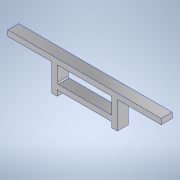
# Autodesk Inventor part: waist1.
Saved by Autodesk Inventor 2022 (Build 260153000, 153)
## iProperties
Created: 2022-10-16
Part Number: waist1.
Material: アルミニウム 6061
Document SubType Name: Modeling
Designer: haya
Density: 2.7 g/cm^3
Appearance: アルミニウム - フラット
Mass: 29.7232 g
Surface Area: 65.8455 cm^2
Volume: 11.0086 cm^3
Author: haya
Autodesk Inventor part; units mm, degrees
ref_plane "YZ Plane" through (0, 0, 0) normal (1, 0, 0) x (0, 1, 0)
ref_plane "XZ Plane" through (0, 0, 0) normal (0, 1, 0) x (-1, 0, 0)
ref_plane "XY Plane" through (0, 0, 0) normal (0, 0, 1) x (1, 0, 0)
sketch "スケッチ1" plane through (0, 0, 0) normal (0, 0, 1) x (1, 0, 0)
  line L0 (130, 25) -> (130, 30)
  line L1 (130, 30) -> (-10, 30)
  line L2 (-10, 30) -> (-10, 25)
  line L3 (60, 30) -> (60, 0) construction
  line L4 (85, 0) -> (85, 5)
  line L5 (85, 5) -> (35, 5)
  line L6 (35, 5) -> (35, 0)
  line L7 (30, 0) -> (35, 0)
  line L8 (85, 0) -> (90, 0)
  line L9 (30, 0) -> (30, 25)
  line L10 (30, 25) -> (-10, 25)
  line L11 (90, 0) -> (90, 25)
  line L12 (90, 25) -> (130, 25)
  dimension "d2" = 50
  dimension "d4" = 5
  dimension "d5" = 5
  dimension "d6" = 5
  dimension "d7" = 140
  dimension "d8" = 30
  constraints: 26 end point, 5 parallel, 2 horizontal, 2 perpendicular, 1 collinear, 1 midpoint, 2 other
  measures "d2" distance of L4.end L5.end
  measures "d4" distance between parallel lines of L8 L5
  measures "d5" distance between parallel lines of L10 L1
  measures "d6" distance between parallel lines of L9 L6
  measures "d7" distance of L0.end L1.end
  measures "d8" distance between parallel lines of L1 L7
extrude "押し出し1" add sketch "スケッチ1" along normal blind 10
sketch "スケッチ2" plane through (0, 0, 0) normal (0, 0, -1) x (-1, 0, 0)
  line L0 (-85, 10) -> (-35, 10)
  line L1 (-35, 10) -> (-35, 25)
  line L2 (-35, 25) -> (-85, 25)
  line L3 (-85, 25) -> (-85, 10)
  line L4 (-90, 0) -> (-90, 25) projected
  line L5 (-85, 0) -> (-90, 0) projected
  line L6 (-85, 5) -> (-85, 0) projected
  line L7 (-35, 5) -> (-85, 5) projected
  line L8 (-35, 0) -> (-35, 5) projected
  line L9 (-30, 0) -> (-35, 0) projected
  line L10 (-30, 25) -> (-30, 0) projected
  line L11 (10, 25) -> (-30, 25) projected
  line L12 (10, 30) -> (10, 25) projected
  line L13 (-130, 30) -> (10, 30) projected
  line L14 (-130, 25) -> (-130, 30) projected
  line L15 (-90, 25) -> (-130, 25) projected
  line L16 (-130, 30) -> (10, 30) projected
  line L17 (-60, 30) -> (-60, 5) construction
  line L18 (-35, 5) -> (-85, 5) projected
  point P0 (0, 0)
  dimension "d11" = 5
  dimension "d12" = 5
  dimension "d13" = 50
  constraints: 10 end point, 2 midpoint, 2 parallel, 1 horizontal, 1 perpendicular, 1 other
  measures "d11" distance between parallel lines of L2 L13
  measures "d12" distance between parallel lines of L7 L0
  measures "d13" distance of L1.end L2.end
extrude "押し出し2" cut sketch "スケッチ2" against normal through all contours L3 L2 L1 L0
fillet "フィレット1" radius 1 4 edges at (85, 25, 5) (35, 25, 5) (35, 10, 5) (85, 10, 5)
